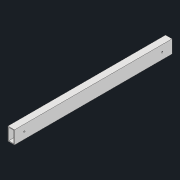
# Autodesk Inventor part: Front Bar
Saved by Autodesk Inventor 2022 (Build 260153000, 153)
## iProperties
Created: 2022-09-10
Part Number: Front Bar
Material: Generic
Document SubType Name: Modeling
Designer: robpl
Density: 1 g/cm^3
Appearance: Default
Author: robpl
Autodesk Inventor part; units mm, degrees
ref_plane "YZ Plane" through (0, 0, 0) normal (1, 0, 0) x (0, 1, 0)
ref_plane "XZ Plane" through (0, 0, 0) normal (0, 1, 0) x (-1, 0, 0)
ref_plane "XY Plane" through (0, 0, 0) normal (0, 0, 1) x (1, 0, 0)
sketch "Sketch1" plane through (0, 0, 0) normal (0, 0, 1) x (1, 0, 0)
  line L0 (0, 0) -> (25, 0)
  line L1 (25, 0) -> (25, 50)
  line L2 (25, 50) -> (0, 50)
  line L3 (0, 50) -> (0, 0)
  line L4 (22, 47) -> (22, 3)
  line L5 (22, 3) -> (3, 3)
  line L6 (3, 3) -> (3, 47)
  line L7 (3, 47) -> (22, 47)
  dimension "d0" = 25
  dimension "d1" = 50
  dimension "d2" = 3
  constraints: 16 end point, 4 parallel, 2 perpendicular, 1 horizontal, 3 other
  measures "d0" distance of L2.end L1.end
  measures "d1" distance of L1.end L0.end
  measures "d2" distance between parallel lines of L1 L4
extrude "Extrusion1" add sketch "Sketch1" along normal blind 600
sketch "Sketch2" plane through (0, 0, 0) normal (1, 0, 0) x (0, 0, -1)
  line L0 (0, 0) -> (-600, 0) projected
  line L1 (-600, 0) -> (-600, 50) projected
  point P0 (-562.5, 25)
  point P1 (-37.5, 25)
  dimension "d5" = 25
  dimension "d6" = 37.5
  dimension "d7" = 37.5
  constraints: 1 horizontal alignment
  measures "d5" distance from line of L0 point (-562.5, 25)
  measures "d6" distance from line of L1 point (-562.5, 25)
  measures "d7" horizontal distance of L0.start point (-37.5, 25)
hole "Hole1" at (0, 25, 562.5) at (0, 25, 37.5) direction (1, 0, 0) diameter 6 end through all counterbore diameter 11 counterbore depth 5
sketch "Sketch3" plane through (0, 0, 0) normal (0, -1, 0) x (1, 0, 0)
  line L0 (0, 0) -> (25, 0) projected
  line L1 (0, 0) -> (0, 600) projected
  point P0 (12.5, 100)
  point P1 (12.5, 200)
  point P2 (12.5, 300)
  point P3 (12.5, 400)
  point P4 (12.5, 500)
  dimension "d15" = 100
  dimension "d16" = 12.5
  dimension "d19" = 100
  constraints: 1 vertical, 4 other
  measures "d15" distance from line of L0 point (12.5, 100)
  measures "d16" distance from line of L1 point (12.5, 100)
  measures "d19" distance of point (12.5, 100) point (12.5, 200)
hole "Hole2" at (12.5, 0, 100) at (12.5, 0, 200) at (12.5, 0, 300) at (12.5, 0, 400) at (12.5, 0, 500) direction (0, 1, 0) diameter 5 depth 8 tip angle 118
body "Solid1"
